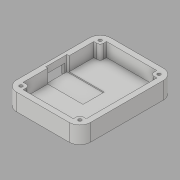
# Autodesk Inventor part: macropad-frame
Saved by Autodesk Inventor 2019 (Build 230136000, 136)
## iProperties
Created: 2019-01-13
Part Number: macropad-frame
Material: Generic
Document SubType Name: Modeling
Designer: onemo
Density: 1 g/cm^3
Appearance: Default
Author: onemo
Autodesk Inventor part; units mm, degrees
ref_plane "YZ Plane" through (0, 0, 0) normal (1, 0, 0) x (0, 1, 0)
ref_plane "XZ Plane" through (0, 0, 0) normal (0, 1, 0) x (-1, 0, 0)
ref_plane "XY Plane" through (0, 0, 0) normal (0, 0, 1) x (1, 0, 0)
sketch "Sketch1" plane through (0, 0, 0) normal (0, 1, 0) x (-1, 0, 0)
  line L0 (40.7087, 37.7886) -> (-28.4413, 37.7886)
  line L1 (-28.4413, 37.7886) -> (-28.4413, -50.4114)
  line L2 (-28.4413, -50.4114) -> (40.7087, -50.4114)
  line L3 (40.7087, -50.4114) -> (40.7087, 37.7886)
  point P0 (0, 0)
  dimension "d0" = 88.2
  dimension "d1" = 69.15
  constraints: 8 end point, 2 parallel, 1 horizontal, 1 perpendicular
  measures "d0" distance between parallel lines of L2 L0
  measures "d1" distance between parallel lines of L1 L3
extrude "Extrusion1" add sketch "Sketch1" along normal blind 3
sketch "Sketch2" plane through (0, 3, 0) normal (0, 1, 0) x (1, 0, 0)
  line L0 (-40.7087, -37.7886) -> (28.4413, -37.7886) projected
  line L1 (28.4413, -37.7886) -> (28.4413, 50.4114) projected
  line L2 (-40.7087, -37.7886) -> (28.4413, -37.7886)
  line L3 (28.4413, -37.7886) -> (28.4413, -32.7886)
  line L4 (28.4413, -32.7886) -> (-40.7087, -32.7886)
  line L5 (-40.7087, -32.7886) -> (-40.7087, -37.7886)
  line L6 (-40.7087, 50.4114) -> (-40.7087, -37.7886) projected
  line L7 (-40.7087, -37.7886) -> (-35.7087, -37.7886)
  line L8 (-35.7087, -37.7886) -> (-35.7087, 50.4114)
  line L9 (-35.7087, 50.4114) -> (-40.7087, 50.4114)
  line L10 (-40.7087, 50.4114) -> (-40.7087, -37.7886)
  line L11 (28.4413, 50.4114) -> (-40.7087, 50.4114) projected
  line L12 (-40.7087, 45.4114) -> (28.4413, 45.4114)
  line L13 (28.4413, 45.4114) -> (28.4413, 50.4114)
  line L14 (28.4413, 50.4114) -> (-40.7087, 50.4114)
  line L15 (-40.7087, 50.4114) -> (-40.7087, 45.4114)
  line L16 (28.4413, 50.4114) -> (23.4413, 50.4114)
  line L17 (23.4413, 50.4114) -> (23.4413, -37.7886)
  line L18 (23.4413, -37.7886) -> (28.4413, -37.7886)
  line L19 (28.4413, -37.7886) -> (28.4413, 50.4114)
  point P0 (0, 0)
  dimension "d4" = 5
  dimension "d5" = 5
  dimension "d6" = 5
  dimension "d7" = 5
  constraints: 32 end point, 8 parallel, 4 horizontal, 4 perpendicular, 3 point on line
  measures "d4" distance between parallel lines of L17 L1
  measures "d5" distance between parallel lines of L0 L4
  measures "d6" distance between parallel lines of L10 L8
  measures "d7" distance between parallel lines of L11 L12
extrude "Extrusion2" add sketch "Sketch2" along normal blind 13 contours L5 L4 L8 L0 | L8 L4 L17 L0 | L6 L12 L8 L4 | L17 L4 L1 L0 | L6 L9 L8 L12 | L17 L12 L1 L4 | L8 L11 L17 L12 | L17 L11 L1 L12
fillet "Fillet1" radius 10 4 edges at (28.4413, 8, 37.7886) (28.4413, 8, -50.4114) (-40.7087, 8, 37.7886) (-40.7087, 8, -50.4114)
sketch "Sketch3" plane through (0, 3, 0) normal (0, 1, 0) x (1, 0, 0)
  line L0 (-35.7087, -32.7886) -> (23.4413, -32.7886) projected
  line L1 (-35.7087, -32.7886) -> (-29.7087, -32.7886)
  line L2 (-29.7087, -32.7886) -> (-29.7087, -26.7886)
  line L3 (-29.7087, -26.7886) -> (-35.7087, -26.7886)
  line L4 (-35.7087, -26.7886) -> (-35.7087, -32.7886)
  line L5 (-35.7087, 45.4114) -> (-35.7087, -32.7886) projected
  line L6 (-35.7087, 45.4114) -> (-29.7087, 45.4114)
  line L7 (-29.7087, 45.4114) -> (-29.7087, 39.4114)
  line L8 (-29.7087, 39.4114) -> (-35.7087, 39.4114)
  line L9 (-35.7087, 39.4114) -> (-35.7087, 45.4114)
  line L10 (23.4413, -32.7886) -> (23.4413, 45.4114) projected
  line L11 (23.4413, 45.4114) -> (17.4413, 45.4114)
  line L12 (17.4413, 45.4114) -> (17.4413, 39.4114)
  line L13 (17.4413, 39.4114) -> (23.4413, 39.4114)
  line L14 (23.4413, 39.4114) -> (23.4413, 45.4114)
  line L15 (23.4413, -32.7886) -> (17.4413, -32.7886)
  line L16 (17.4413, -32.7886) -> (17.4413, -26.7886)
  line L17 (17.4413, -26.7886) -> (23.4413, -26.7886)
  line L18 (23.4413, -26.7886) -> (23.4413, -32.7886)
  point P0 (0, 0)
  dimension "d11" = 6
  dimension "d12" = 6
  dimension "d13" = 6
  dimension "d14" = 6
  dimension "d15" = 6
  dimension "d16" = 6
  dimension "d17" = 6
  dimension "d18" = 6
  constraints: 32 end point, 8 parallel, 4 horizontal, 4 perpendicular
  measures "d11" distance between parallel lines of L3 L0
  measures "d12" distance between parallel lines of L4 L2
  measures "d13" distance between parallel lines of L6 L8
  measures "d14" distance between parallel lines of L5 L7
  measures "d15" distance between parallel lines of L13 L11
  measures "d16" distance between parallel lines of L12 L10
  measures "d17" distance between parallel lines of L17 L15
  measures "d18" distance between parallel lines of L16 L10
extrude "Extrusion3" add sketch "Sketch3" along normal up to surface (13 mm away)
fillet "Fillet2" radius 3 4 edges at (-29.7087, 9.5, -39.4114) (-29.7087, 9.5, 26.7886) (17.4413, 9.5, -39.4114) (17.4413, 9.5, 26.7886)
sketch "Sketch4" plane through (0, 16, 0) normal (0, 1, 0) x (1, 0, 0)
  line L0 (28.4413, -27.7886) -> (28.4413, 40.4114) projected
  line L1 (-30.7087, -37.7886) -> (18.4413, -37.7886) projected
  line L2 (-40.7087, 40.4114) -> (-40.7087, -27.7886) projected
  line L3 (18.4413, 50.4114) -> (-30.7087, 50.4114) projected
  point P0 (0, 0)
  point P1 (21.4413, -30.7886)
  point P2 (-33.7087, -30.7886)
  point P3 (-33.7087, 43.4114)
  point P4 (21.4413, 43.4114)
  dimension "d22" = 7
  dimension "d23" = 7
  dimension "d24" = 7
  dimension "d25" = 7
  dimension "d26" = 7
  dimension "d27" = 7
  dimension "d28" = 7
  dimension "d29" = 7
  measures "d22" distance from line of L0 point (21.441, -30.789)
  measures "d23" distance from line of L1 point (21.441, -30.789)
  measures "d24" distance from line of L1 point (-33.709, -30.789)
  measures "d25" distance from line of L2 point (-33.709, -30.789)
  measures "d26" distance from line of L2 point (-33.709, 43.411)
  measures "d27" distance from line of point (-33.709, 43.411) L3
  measures "d28" distance from line of L3 point (21.441, 43.411)
  measures "d29" distance from line of point (21.441, 43.411) L0
hole "Hole1" at (21.4413, 16, 30.7886) at (-33.7087, 16, 30.7886) at (-33.7087, 16, -43.4114) at (21.4413, 16, -43.4114) direction (0, -1, 0) diameter 3 depth 6
sketch "Sketch5" plane through (-35.7087, 3, 26.7886) normal (1, 0, 0) x (0, 0, -1)
  line L0 (66.2, 0) -> (0, 0) projected
  line L1 (28, 0) -> (38.2, 0)
  line L2 (38.2, 0) -> (38.2, 4)
  line L3 (38.2, 4) -> (28, 4)
  line L4 (28, 4) -> (28, 0)
  line L5 (0, 13) -> (0, 0) projected
  point P0 (26.7886, -3)
  point P1 (66.2, 13)
  dimension "d37" = 4
  dimension "d38" = 10.2
  dimension "d39" = 28
  dimension "d40" = 28
  dimension "d41" = 66.2
  constraints: 8 end point, 2 parallel, 1 horizontal, 1 perpendicular, 1 point on line
  measures "d37" distance between parallel lines of L3 L0
  measures "d38" distance between parallel lines of L2 L4
  measures "d39" distance from line of point (66.2, 13) L2
  measures "d40" distance between parallel lines of L5 L4
  measures "d41" distance of L0.start L0.end
extrude "Extrusion4" cut sketch "Sketch5" against normal blind 13
sketch "Sketch6" plane through (-40.7087, 0, -40.4114) normal (-1, 0, 0) x (0, 0, 1)
  line L0 (26, 10) -> (42.2, 10)
  line L1 (42.2, 10) -> (42.2, 0)
  line L2 (42.2, 0) -> (26, 0)
  line L3 (26, 0) -> (26, 10)
  line L4 (39.2, 7) -> (39.2, 3) projected
  line L5 (29, 3) -> (29, 7) projected
  line L6 (39.2, 3) -> (29, 3) projected
  line L7 (29, 7) -> (39.2, 7) projected
  point P0 (40.4114, 0)
  dimension "d44" = 3
  dimension "d45" = 3
  dimension "d46" = 3
  dimension "d47" = 3
  constraints: 8 end point, 2 parallel, 1 horizontal, 1 perpendicular
  measures "d44" distance between parallel lines of L1 L4
  measures "d45" distance between parallel lines of L3 L5
  measures "d46" distance between parallel lines of L6 L2
  measures "d47" distance between parallel lines of L0 L7
extrude "Extrusion5" cut sketch "Sketch6" against normal blind 3
sketch "Sketch7" plane through (-35.7087, 3, -39.4114) normal (1, 0, 0) x (0, 0, -1)
  line L0 (-38.2, 0) -> (-66.2, 0) projected
  line L1 (-43.1, 0) -> (-23.1, 0)
  line L2 (-23.1, 0) -> (-23.1, 300)
  line L3 (-23.1, 300) -> (-43.1, 300)
  line L4 (-43.1, 300) -> (-43.1, 0)
  line L5 (-28, 4) -> (-28, 0) projected
  line L6 (-38.2, 0) -> (-38.2, 4) projected
  point P0 (-39.4114, -3)
  dimension "d50" = 20
  dimension "d51" = 4.9
  dimension "d52" = 4.9
  dimension "d53" = 10.2
  dimension "d102" = 300
  constraints: 8 end point, 2 parallel, 1 horizontal, 1 perpendicular, 1 point on line
  measures "d50" distance between parallel lines of L2 L4
  measures "d51" distance between parallel lines of L5 L2
  measures "d52" distance between parallel lines of L4 L6
  measures "d53" distance between parallel lines of L5 L6
  measures "d102" distance between parallel lines of L3 L1
extrude "Extrusion6" cut sketch "Sketch7" against normal blind 2
sketch "Sketch8" plane through (0, 3, 0) normal (0, 1, 0) x (1, 0, 0)
  line L0 (-37.7087, 16.3114) -> (-37.7087, 14.4114) projected
  line L1 (-37.7087, 16.3114) -> (-2.7087, 16.3114)
  line L2 (-2.7087, 16.3114) -> (-2.7087, -3.6886)
  line L3 (-2.7087, -3.6886) -> (-37.7087, -3.6886)
  line L4 (-37.7087, -3.6886) -> (-37.7087, 16.3114)
  line L5 (-35.7087, -3.6886) -> (-37.7087, -3.6886) projected
  point P0 (0, 0)
  dimension "d56" = 20
  dimension "d57" = 20
  dimension "d58" = 35
  constraints: 8 end point, 2 parallel, 1 horizontal, 1 perpendicular
  measures "d56" distance of L3.end L0.start
  measures "d57" distance between parallel lines of L1 L5
  measures "d58" distance between parallel lines of L2 L4
extrude "Extrusion7" cut sketch "Sketch8" against normal blind 1
sketch "Sketch14" plane through (0, 3, 0) normal (0, 1, 0) x (1, 0, 0)
  line L0 (-27.7087, -26.7886) -> (-21.5087, -26.7886)
  line L1 (-21.5087, -26.7886) -> (-21.5087, -20.5886)
  line L2 (-21.5087, -20.5886) -> (-27.7087, -20.5886)
  line L3 (-27.7087, -20.5886) -> (-27.7087, -26.7886)
  line L4 (17.4413, -32.7886) -> (-29.7087, -32.7886) projected
  line L5 (-35.7087, -26.7886) -> (-35.7087, -3.6886) projected
  point P0 (0, 0)
  dimension "d103" = 6.2
  dimension "d104" = 6
  dimension "d105" = 8
  dimension "d106" = 6.2
  constraints: 8 end point, 2 parallel, 1 horizontal, 1 perpendicular
  measures "d103" distance between parallel lines of L2 L0
  measures "d104" distance between parallel lines of L4 L0
  measures "d105" distance between parallel lines of L5 L3
  measures "d106" distance between parallel lines of L3 L1
extrude "Extrusion11" cut sketch "Sketch14" against normal blind 1
sketch "Sketch15" plane through (0, 2, 0) normal (0, 1, 0) x (1, 0, 0)
  circle A0 centre (-24.6087, -23.6886) radius 1.875
  line L0 (-21.5087, -20.5886) -> (-21.5087, -26.7886) projected
  line L1 (-27.7087, -26.7886) -> (-27.7087, -20.5886) projected
  line L2 (-27.7087, -20.5886) -> (-21.5087, -20.5886) projected
  line L3 (-21.5087, -26.7886) -> (-27.7087, -26.7886) projected
  point P0 (0, 0)
  dimension "d109" = 3.1
  dimension "d110" = 3.1
  dimension "d111" = 3.1
  dimension "d112" = 3.1
  dimension "d113" = 3.75
  constraints: 1 centre point
  measures "d109" distance from line of L0 A0.centre
  measures "d110" distance from line of L1 A0.centre
  measures "d111" distance from line of L2 A0.centre
  measures "d112" distance from line of L3 A0.centre
  measures "d113" diameter of A0
extrude "Extrusion12" cut sketch "Sketch15" against normal through all contours A0
equation "\"d5\" = d4"
equation "\"d6\" = d4"
equation "\"d7\" = d4"
equation "\"d11\" = d12"
equation "\"d13\" = d12"
equation "\"d14\" = d13"
equation "\"d15\" = d13"
equation "\"d16\" = d15"
equation "\"d17\" = d15"
equation "\"d18\" = d17"
equation "\"d22\" = d23"
equation "\"d24\" = d23"
equation "\"d25\" = d24"
equation "\"d26\" = d25"
equation "\"d27\" = d26"
equation "\"d28\" = d27"
equation "\"d29\" = d28"
equation "\"d39\" = 0.5 * d41 - 0.5 * d38"
equation "\"d45\" = d44"
equation "\"d47\" = d44"
equation "\"d51\" = -0.5 * d53 + 0.5 * d50"
equation "\"d56\" = d57"
equation "\"d103\" = d106"
equation "\"d109\" = d112"
body "Solid1"
